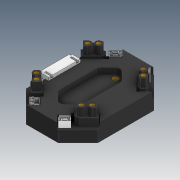
# Autodesk Inventor part: terminal_board
Saved by Autodesk Inventor 2020 (Build 240168000, 168)
## iProperties
Created: 2020-09-28
Part Number: terminal_board
Material: Generic
Document SubType Name: Modeling
Designer: DELL
Density: 1 g/cm^3
Appearance: White
Author: DELL
Autodesk Inventor part; units mm, degrees
ref_plane "YZ Plane" through (0, 0, 0) normal (1, 0, 0) x (0, 1, 0)
ref_plane "XZ Plane" through (0, 0, 0) normal (0, 1, 0) x (-1, 0, 0)
ref_plane "XY Plane" through (0, 0, 0) normal (0, 0, 1) x (1, 0, 0)
sketch "Sketch1" plane through (0, 0, 0) normal (0, 1, 0) x (-1, 0, 0)
  line L0 (22.5, 17.5) -> (22.5, -17.5)
  line L1 (22.5, -17.5) -> (10, -30)
  line L2 (10, -30) -> (-10, -30)
  line L3 (-10, -30) -> (-22.5, -17.5)
  line L4 (-22.5, -17.5) -> (-22.5, 17.5)
  line L5 (-22.5, 17.5) -> (-10, 30)
  line L6 (-10, 30) -> (10, 30)
  line L7 (10, 30) -> (22.5, 17.5)
  line L8 (30.1038, 0) -> (-31.33, 0) construction
  line L9 (0, 32.2243) -> (0, -47.739) construction
  point P0 (0, 0)
  dimension "d0" = 45
  dimension "d1" = 60
  dimension "d2" = 20
  dimension "d3" = 35
  constraints: 20 end point, 2 horizontal, 2 point on line, 2 vertical, 1 parallel, 1 perpendicular, 5 other
  measures "d0" distance between parallel lines of L4 L0
  measures "d1" distance between parallel lines of L2 L6
  measures "d2" distance of L1.end L2.end
  measures "d3" distance of L0.start L0.end
extrude "Extrusion1" add sketch "Sketch1" along normal blind 6.8
sketch "Sketch2" plane through (0, 6.8, 0) normal (0, 1, 0) x (1, 0, 0)
  line L0 (-21.4393, 15.7322) -> (-15.4289, 21.7426)
  line L1 (-15.4289, 21.7426) -> (-11.6813, 17.995)
  line L2 (-11.6813, 17.995) -> (-17.6917, 11.9846)
  line L3 (-17.6917, 11.9846) -> (-21.4393, 15.7322)
  line L4 (-10, 30) -> (-22.5, 17.5) projected
  line L5 (-15.4289, 21.7426) -> (-12.6712, 22.5205)
  line L6 (-12.6712, 22.5205) -> (-10.9034, 20.7527)
  line L7 (-10.9034, 20.7527) -> (-11.6813, 17.995)
  line L8 (-19.5655, 13.8584) -> (-13.5551, 19.8688) construction
  point P0 (0, 0)
  dimension "d6" = 5.3
  dimension "d7" = 11
  dimension "d8" = 8.5
  dimension "d9" = 2.5
  dimension "d10" = 2
  dimension "d11" = 0.5
  constraints: 17 end point, 3 perpendicular, 2 midpoint, 1 parallel, 1 other
  measures "d6" distance between parallel lines of L2 L0
  measures "d7" distance between parallel lines of L3 L6
  measures "d8" distance between parallel lines of L3 L1
  measures "d9" distance of L5.end L6.end
  measures "d10" distance between parallel lines of L4 L0
  measures "d11" distance from line of L4.end L3
extrude "Extrusion2" add sketch "Sketch2" along normal blind 5.2
sketch "Sketch3" plane through (0, 12, 0) normal (0, 1, 0) x (1, 0, 0)
  line L0 (-10.9034, 20.7527) -> (-12.6712, 22.5205) projected
  line L1 (-12.6712, 22.5205) -> (-15.4289, 21.7426) projected
  line L2 (-15.4289, 21.7426) -> (-21.4393, 15.7322) projected
  line L3 (-21.4393, 15.7322) -> (-17.6917, 11.9846) projected
  line L4 (-17.6917, 11.9846) -> (-11.6813, 17.995) projected
  line L5 (-11.6813, 17.995) -> (-10.9034, 20.7527) projected
  line L6 (-14.5509, 21.4708) -> (-13.3632, 21.8058)
  circle A0 centre (-17.3735, 16.0504) radius 1.25
  circle A1 centre (-13.9794, 19.4445) radius 1.25
  line L7 (-19.212, 14.212) -> (-12.1409, 21.283) construction
  line L8 (-17.1967, 19.2678) -> (-14.1561, 16.2272) construction
  line L9 (-17.3735, 13.0731) -> (-15.8848, 14.5618)
  line L10 (-17.3735, 13.0731) -> (-20.3508, 16.0504)
  line L11 (-13.3632, 21.8058) -> (-11.6181, 20.0607)
  line L12 (-10.9034, 20.7527) -> (-12.6712, 22.5205) projected
  line L13 (-15.7186, 17.3518) -> (-15.2807, 17.7896)
  line L14 (-16.0721, 17.7053) -> (-15.6343, 18.1432)
  line L15 (-11.6181, 20.0607) -> (-11.9531, 18.873)
  line L16 (-20.3508, 16.0504) -> (-18.8621, 17.5391)
  arc A2 (-15.8848, 14.5618) -> (-15.7186, 17.3518) centre (-17.3735, 16.0504) ccw
  arc A3 (-16.0721, 17.7053) -> (-18.8621, 17.5391) centre (-17.3735, 16.0504) ccw
  arc A4 (-14.5509, 21.4708) -> (-15.6343, 18.1432) centre (-13.9794, 19.4445) ccw
  arc A5 (-15.2807, 17.7896) -> (-11.9531, 18.873) centre (-13.9794, 19.4445) ccw
  point P0 (0, 0)
  dimension "d15" = 4.8
  dimension "d16" = 2.5
  dimension "d17" = 0.5
  constraints: 20 end point, 8 point on circle, 6 centre point, 5 tangent, 2 coincident, 2 parallel, 2 point on line, 1 equal radius, 1 symmetric about line, 1 other
  measures "d15" distance of A1.centre A0.centre
  measures "d16" diameter of A0
  measures "d17" distance between parallel lines of L13 L14
extrude "Extrusion3" add sketch "Sketch3" along normal blind 5.2 contours L6 L11 L15 A5 L13 A2 L9 L10 L16 A3 L14 A4
sketch "Sketch4" plane through (0, 6.8, 0) normal (0, 1, 0) x (1, 0, 0)
  line L0 (-15.7186, 17.3518) -> (-15.2807, 17.7896) projected
  line L1 (-15.4996, 17.5707) -> (0, 2.0711)
  line L2 (0, 0) -> (0, 30.0261)
  constraints: 4 end point, 1 coincident, 1 midpoint, 1 perpendicular, 1 point on line, 1 vertical
fillet "Fillet1" radius 0.2 4 edges at (-15.7186, 14.6, -17.3518) (-15.2807, 14.6, -17.7896) (-16.0721, 14.6, -17.7053) (-15.6343, 14.6, -18.1432)
fillet "Fillet2" radius 0.2 2 edges at (-11.6181, 14.6, -20.0607) (-13.3632, 14.6, -21.8058)
pattern_circular "Circular Pattern1" count 2 over 270 about axis through (0, 6.8, -2.0711) along (0, 1, 0) of "Extrusion2", "Extrusion3", "Fillet1", "Fillet2"
pattern_circular "Circular Pattern2" count 2 over 360 about axis through (0, -10, 0) along (0, 1, 0) of "Extrusion2", "Extrusion3", "Fillet1", "Fillet2", "Circular Pattern1"
sketch "Sketch5" plane through (0, 6.8, 0) normal (0, 1, 0) x (1, 0, 0)
  line L0 (-13.0406, 24.8381) -> (-9.8586, 21.6561)
  line L1 (-9.8586, 21.6561) -> (-5.7574, 25.7574)
  line L2 (-5.7574, 25.7574) -> (-8.9393, 28.9393)
  line L3 (-8.9393, 28.9393) -> (-13.0406, 24.8381)
  line L4 (-10, 30) -> (-22.5, 17.5) projected
  line L5 (10, 30) -> (-10, 30) projected
  point P0 (0, 0)
  point P1 (-10, 30)
  dimension "d28" = 1.5
  dimension "d29" = 5.8
  dimension "d30" = 4.5
  constraints: 8 end point, 2 parallel, 2 perpendicular, 1 coincident, 1 point on line
  measures "d28" distance between parallel lines of L4 L3
  measures "d29" distance of L2.end L0.start
  measures "d30" distance of L1.end L2.end
extrude "Extrusion4" add sketch "Sketch5" along normal blind 4.15
sketch "Sketch6" plane through (0, 10.95, 0) normal (0, 1, 0) x (1, 0, 0)
  line L0 (-12.6163, 24.8381) -> (-12.192, 24.4139)
  line L1 (-12.192, 24.4139) -> (-11.4849, 25.121)
  line L2 (-11.4849, 25.121) -> (-11.9092, 25.5452)
  line L3 (-11.9092, 25.5452) -> (-12.6163, 24.8381)
  line L4 (-8.9393, 28.9393) -> (-13.0406, 24.8381) projected
  line L5 (-13.0406, 24.8381) -> (-9.8586, 21.6561) projected
  line L6 (-13.0406, 24.8381) -> (-8.9393, 28.9393) construction
  line L7 (-10.9899, 26.8887) -> (-7.808, 23.7067) construction
  line L8 (-8.9393, 28.5151) -> (-8.5151, 28.0908)
  line L9 (-8.5151, 28.0908) -> (-9.2222, 27.3837)
  line L10 (-9.2222, 27.3837) -> (-9.6464, 27.808)
  line L11 (-9.6464, 27.808) -> (-8.9393, 28.5151)
  line L12 (-11.5556, 25.8988) -> (-10.4243, 24.7674)
  line L13 (-10.4243, 24.7674) -> (-8.8686, 26.323)
  line L14 (-8.8686, 26.323) -> (-10, 27.4544)
  line L15 (-10, 27.4544) -> (-11.5556, 25.8988)
  line L16 (-5.7574, 25.7574) -> (-8.9393, 28.9393) construction
  line L17 (-8.9393, 28.9393) -> (-13.0406, 24.8381) construction
  line L18 (-13.0406, 24.8381) -> (-9.8586, 21.6561) construction
  line L19 (-9.8586, 21.6561) -> (-5.7574, 25.7574) construction
  line L20 (-8.9393, 28.5151) -> (-12.6163, 24.8381) construction
  line L21 (-9.6464, 22.2925) -> (-6.3938, 25.5452)
  line L22 (-11.7678, 24.4139) -> (-11.1314, 25.0503)
  line L23 (-11.1314, 25.0503) -> (-10.4243, 24.3431)
  line L24 (-10.4243, 24.3431) -> (-8.4444, 26.323)
  line L25 (-8.4444, 26.323) -> (-9.1515, 27.0302)
  line L26 (-9.1515, 27.0302) -> (-8.5151, 27.6665)
  line L27 (-12.6163, 24.8381) -> (-12.192, 24.4139)
  line L28 (-11.7678, 24.4139) -> (-9.6464, 22.2925)
  line L29 (-6.3938, 25.5452) -> (-8.5151, 27.6665)
  line L30 (-8.5151, 28.0908) -> (-8.9393, 28.5151)
  point P0 (0, 0)
  dimension "d34" = 0.3
  dimension "d35" = 0.3
  dimension "d36" = 1
  dimension "d37" = 0.6
  dimension "d40" = 2.2
  dimension "d41" = 1.6
  dimension "d42" = 0.3
  dimension "d43" = 0.3
  dimension "d45" = 0.3
  dimension "d46" = 0.3
  dimension "d47" = 0.3
  dimension "d48" = 0.6
  dimension "d49" = 0.6
  dimension "d50" = 0.3
  constraints: 48 end point, 10 perpendicular, 4 symmetric about line, 2 point on line, 1 midpoint, 1 parallel, 1 other
  measures "d34" distance between parallel lines of L4 L3
  measures "d35" distance between parallel lines of L5 L0
  measures "d36" distance of L0.end L1.end
  measures "d37" distance of L0.start L0.end
  measures "d40" distance of L14.end L12.start
  measures "d41" distance of L12.start L12.end
  measures "d42" distance between parallel lines of L4 L15
  measures "d43" distance between parallel lines of L12 L23
  measures "d45" distance between parallel lines of L13 L24
  measures "d46" distance between parallel lines of L14 L25
  measures "d47" distance between parallel lines of L9 L26
  measures "d48" distance between parallel lines of L5 L28
  measures "d49" distance between parallel lines of L16 L29
  measures "d50" distance between parallel lines of L19 L21
extrude "Extrusion5" cut sketch "Sketch6" against normal up to surface (4.15 mm away) contours L3 L2 L1 L0 | L8 L9 L10 L11 | L15 L14 L13 L12
extrude "Extrusion6" cut sketch "Sketch6" against normal blind 3 contours L28 L22 L23 L24 L25 L26 L29 L21
sketch "Sketch7" plane through (-8.9393, 6.8, -28.9393) normal (0.7071068, 0, -0.7071068) x (-0.7071068, 0, -0.7071068)
  line L0 (-4.5, 4.15) -> (0, 4.15) projected
  line L1 (-1.9, 4.15) -> (-4.5, 4.15)
  line L2 (-4.5, 4.15) -> (-4.5, 1.8317)
  line L3 (-4.5, 0) -> (-4.5, 4.15) projected
  line L4 (-4.5, 1.8317) -> (-3.7, 1.8317)
  line L5 (-3.7, 1.8317) -> (-3.7, 3.55)
  line L6 (-3.7, 3.55) -> (-1.9, 3.55)
  line L7 (-1.9, 4.15) -> (-1.9, 0) projected
  line L8 (-1.9, 3.55) -> (-1.9, 4.15)
  point P0 (-26.7843, -6.8)
  dimension "d55" = 0.6
  dimension "d56" = 0.8
  constraints: 12 end point, 3 perpendicular, 3 point on line, 1 collinear, 1 horizontal
  measures "d55" distance between parallel lines of L0 L6
  measures "d56" distance between parallel lines of L5 L2
extrude "Extrusion7" cut sketch "Sketch7" against normal blind 0.3
ref_plane "Work Plane1" through (-10.9899, 6.8, -26.8887) normal (0.7071068, 0, -0.7071068) x (-0.7071068, 0, -0.7071068)
mirror "Mirror1" about plane through (-10.9899, 6.8, -26.8887) normal (0.7071068, 0, -0.7071068) of "Extrusion7"
sketch "Sketch8" plane through (0, 6.8, 0) normal (0, 1, 0) x (1, 0, 0)
  line L0 (0, 0) -> (0, 30)
  line L1 (10, 30) -> (-10, 30) projected
  line L2 (-8.9393, 28.9393) -> (-13.0406, 24.8381) projected
  line L3 (-10.9899, 26.8887) -> (0, 15.8988)
  constraints: 4 end point, 2 midpoint, 1 coincident, 1 perpendicular, 1 point on line
pattern_circular "Circular Pattern3" count 2 over 270 about axis through (0, 6.8, -15.8988) along (0, 1, 0) of "Extrusion6", "Extrusion4", "Extrusion5", "Extrusion7", "Mirror1"
pattern_circular "Circular Pattern4" count 2 over 360 about axis through (0, -10, 0) along (0, 1, 0) of "Extrusion4", "Extrusion5", "Extrusion6", "Extrusion7", "Mirror1", "Circular Pattern3"
sketch "Sketch9" plane through (0, 6.8, 0) normal (0, 1, 0) x (1, 0, 0)
  line L0 (-16, -10) -> (-22, -10)
  line L1 (-22, -10) -> (-22, 10)
  line L2 (-22, 10) -> (-16, 10)
  line L3 (-16, 10) -> (-16, -10)
  line L4 (-16, -10) -> (-22, 10) construction
  line L5 (-22, -10) -> (-16, 10) construction
  line L6 (-22.5, 17.5) -> (-22.5, -17.5) projected
  line L7 (-22.5, 0) -> (22.5, 0) construction
  line L8 (22.5, -17.5) -> (22.5, 17.5) construction
  point P0 (0, 0)
  point P1 (-19, 0)
  point P2 (-19, 0)
  dimension "d65" = 20
  dimension "d66" = 6
  dimension "d67" = 0.5
  constraints: 14 end point, 5 midpoint, 2 parallel, 1 horizontal, 1 perpendicular, 1 point on line
  measures "d65" distance of L0.end L1.end
  measures "d66" distance of L1.end L2.end
  measures "d67" distance between parallel lines of L6 L1
extrude "Extrusion8" add sketch "Sketch9" along normal blind 5.6
sketch "Sketch10" plane through (-22, 6.8, -10) normal (-1, 0, 0) x (0, 0, 1)
  line L0 (20, 0) -> (0, 0) projected
  line L1 (20, 0) -> (20, 5.6) projected
  line L2 (0, 5.6) -> (20, 5.6) projected
  line L3 (0, 0) -> (0, 5.6) projected
  line L4 (19.5, 4.36) -> (19.5, 0.5)
  line L5 (19.5, 0.5) -> (0.5, 0.5)
  line L6 (0.5, 0.5) -> (0.5, 4.36)
  line L7 (4, 5.1) -> (16, 5.1)
  line L8 (0.5, 4.36) -> (0.5, 0.5)
  line L9 (0.5, 0.5) -> (19.5, 0.5)
  line L10 (19.5, 0.5) -> (19.5, 4.36)
  line L11 (19.5, 4.36) -> (0.5, 0.5) construction
  line L12 (0.5, 4.36) -> (19.5, 0.5) construction
  line L13 (4, 4.36) -> (4, 5.1)
  line L14 (4, 5.1) -> (16, 5.1)
  line L15 (16, 5.1) -> (16, 4.36)
  line L16 (16, 4.36) -> (4, 5.1) construction
  line L17 (4, 4.36) -> (16, 5.1) construction
  line L18 (19.5, 4.36) -> (16, 4.36)
  line L19 (4, 4.36) -> (0.5, 4.36)
  point P0 (10, -6.8)
  point P1 (10, 2.43)
  point P2 (10, 4.73)
  point P3 (10, 4.73)
  point P4 (10, 2.43)
  dimension "d70" = 0.5
  dimension "d72" = 12
  dimension "d73" = 3.86
  dimension "d74" = 19
  dimension "d75" = 0.5
  dimension "d76" = 4.36
  constraints: 32 end point, 6 midpoint, 4 parallel, 3 collinear, 2 horizontal, 2 perpendicular, 1 vertical alignment
  measures "d70" distance between parallel lines of L2 L7
  measures "d72" distance of L7.start L7.end
  measures "d73" distance between parallel lines of L5 L19
  measures "d74" distance between parallel lines of L4 L6
  measures "d75" distance between parallel lines of L3 L6
  measures "d76" distance between parallel lines of L0 L19
extrude "Extrusion9" cut sketch "Sketch10" against normal blind 5.6 contours L4 L5 L6 L19 L13 L7 L15 L18
sketch "Sketch11" plane through (0, 12.4, 0) normal (0, 1, 0) x (1, 0, 0)
  line L0 (-16, 8.5) -> (-20, 8.5)
  line L1 (-20, 8.5) -> (-20, 7.5)
  line L2 (-20, 7.5) -> (-16, 7.5)
  line L3 (-16, 7.5) -> (-16, 8.5)
  line L4 (-16, 10) -> (-16, -10) projected
  line L5 (-16, -7.5) -> (-20, -7.5)
  line L6 (-20, -7.5) -> (-20, -8.5)
  line L7 (-20, -8.5) -> (-16, -8.5)
  line L8 (-16, -8.5) -> (-16, -7.5)
  line L9 (-16, 10) -> (-22, 10) projected
  line L10 (-22, 10) -> (-22, -10) projected
  line L11 (-16, 0) -> (-22, 0) construction
  line L12 (-22, 6) -> (-22, -6) construction
  point P0 (0, 0)
  dimension "d79" = 1
  dimension "d80" = 1.5
  dimension "d81" = 2
  constraints: 18 end point, 4 parallel, 2 horizontal, 2 midpoint, 2 perpendicular, 2 point on line, 2 other
  measures "d79" distance of L0.end L1.end
  measures "d80" distance between parallel lines of L9 L0
  measures "d81" distance between parallel lines of L10 L1
extrude "Extrusion10" cut sketch "Sketch11" against normal up to surface (1.24 mm away)
sketch "Sketch12" plane through (0, 12.4, 0) normal (0, 1, 0) x (1, 0, 0)
  line L0 (-16, 10) -> (-22, 10) projected
  line L1 (-22, 10) -> (-21, 10)
  line L2 (-21, 10) -> (-21, 9)
  line L3 (-21, 9) -> (-22, 9)
  line L4 (-22, 9) -> (-22, 10)
  line L5 (-22, -10) -> (-16, -10) projected
  line L6 (-22, -10) -> (-21, -10)
  line L7 (-21, -10) -> (-21, -9)
  line L8 (-21, -9) -> (-22, -9)
  line L9 (-22, -9) -> (-22, -10)
  point P0 (0, 0)
  dimension "d84" = 1
  dimension "d85" = 1
  dimension "d86" = 1
  dimension "d87" = 1
  constraints: 16 end point, 4 parallel, 2 horizontal, 2 perpendicular
  measures "d84" distance of L2.end L3.end
  measures "d85" distance of L1.end L2.end
  measures "d86" distance of L7.end L8.end
  measures "d87" distance of L6.end L7.end
extrude "Extrusion11" cut sketch "Sketch12" against normal up to surface (5.6 mm away)
sketch "Sketch13" plane through (-21, 12.4, 9) normal (-1, 0, 0) x (0, 0, 1)
  line L0 (-19, -5.6) -> (-19, 0) projected
  line L1 (1, -2.5) -> (-19, -2.5)
  line L2 (-19, -2.5) -> (-19, -2)
  line L3 (-19, -2) -> (1, -2)
  line L4 (1, -2) -> (1, -2.5)
  line L5 (1, -2.5) -> (-19, -2) construction
  line L6 (-19, -2.5) -> (1, -2) construction
  line L7 (-18, 0) -> (0, 0) projected
  line L8 (1, 0) -> (1, -5.6) projected
  point P0 (-9, -12.4)
  point P1 (-9, -2.25)
  dimension "d90" = 2
  dimension "d91" = 0.5
  constraints: 12 end point, 2 midpoint, 2 parallel, 1 collinear, 1 horizontal, 1 perpendicular, 1 point on line
  measures "d90" distance between parallel lines of L7 L3
  measures "d91" distance between parallel lines of L1 L3
extrude "Extrusion12" cut sketch "Sketch13" against normal blind 1.5
sketch "Sketch14" plane through (0, 6.8, 0) normal (0, 1, 0) x (1, 0, 0)
  line L0 (-16, -10) -> (-21, -10) projected
  line L1 (-21, -9) -> (-21, -10) projected
  line L2 (-22, -9) -> (-21, -9) projected
  line L3 (-22, -9) -> (-22, 9) projected
  line L4 (-21, 9) -> (-22, 9) projected
  line L5 (-21, 10) -> (-21, 9) projected
  line L6 (-21, 10) -> (-16, 10) projected
  line L7 (-16, 10) -> (-16, -10) projected
  line L8 (-5.7574, -25.7574) -> (-8.9393, -28.9393) projected
  line L9 (-8.9393, -28.9393) -> (-13.0406, -24.8381) projected
  line L10 (-13.0406, -24.8381) -> (-9.8586, -21.6561) projected
  line L11 (-9.8586, -21.6561) -> (-5.7574, -25.7574) projected
  line L12 (9.8586, -21.6561) -> (13.0406, -24.8381) projected
  line L13 (13.0406, -24.8381) -> (8.9393, -28.9393) projected
  line L14 (8.9393, -28.9393) -> (5.7574, -25.7574) projected
  line L15 (5.7574, -25.7574) -> (9.8586, -21.6561) projected
  line L16 (5.7574, 25.7574) -> (8.9393, 28.9393) projected
  line L17 (8.9393, 28.9393) -> (13.0406, 24.8381) projected
  line L18 (13.0406, 24.8381) -> (9.8586, 21.6561) projected
  line L19 (9.8586, 21.6561) -> (5.7574, 25.7574) projected
  line L20 (-9.8586, 21.6561) -> (-13.0406, 24.8381) projected
  line L21 (-13.0406, 24.8381) -> (-8.9393, 28.9393) projected
  line L22 (-8.9393, 28.9393) -> (-5.7574, 25.7574) projected
  line L23 (-5.7574, 25.7574) -> (-9.8586, 21.6561) projected
  line L24 (-9.9135, -19.7627) -> (-13.6612, -23.5104) projected
  line L25 (-13.6612, -23.5104) -> (-19.6716, -17.5) projected
  line L26 (-19.6716, -17.5) -> (-20.4494, -14.7423) projected
  line L27 (-20.4494, -14.7423) -> (-18.6816, -12.9745) projected
  line L28 (-18.6816, -12.9745) -> (-15.9239, -13.7523) projected
  line L29 (-15.9239, -13.7523) -> (-9.9135, -19.7627) projected
  line L30 (17.6917, -11.9846) -> (21.4393, -15.7322) projected
  line L31 (21.4393, -15.7322) -> (15.4289, -21.7426) projected
  line L32 (15.4289, -21.7426) -> (12.6712, -22.5205) projected
  line L33 (12.6712, -22.5205) -> (10.9034, -20.7527) projected
  line L34 (10.9034, -20.7527) -> (11.6813, -17.995) projected
  line L35 (11.6813, -17.995) -> (17.6917, -11.9846) projected
  line L36 (9.9135, 19.7627) -> (13.6612, 23.5104) projected
  line L37 (13.6612, 23.5104) -> (19.6716, 17.5) projected
  line L38 (19.6716, 17.5) -> (20.4494, 14.7423) projected
  line L39 (20.4494, 14.7423) -> (18.6816, 12.9745) projected
  line L40 (18.6816, 12.9745) -> (15.9239, 13.7523) projected
  line L41 (15.9239, 13.7523) -> (9.9135, 19.7627) projected
  line L42 (-17.6917, 11.9846) -> (-21.4393, 15.7322) projected
  line L43 (-21.4393, 15.7322) -> (-15.4289, 21.7426) projected
  line L44 (-15.4289, 21.7426) -> (-12.6712, 22.5205) projected
  line L45 (-12.6712, 22.5205) -> (-10.9034, 20.7527) projected
  line L46 (-10.9034, 20.7527) -> (-11.6813, 17.995) projected
  line L47 (-11.6813, 17.995) -> (-17.6917, 11.9846) projected
  line L48 (-10, -30) -> (10, -30) projected
  line L49 (10, -30) -> (22.5, -17.5) projected
  line L50 (22.5, -17.5) -> (22.5, 17.5) projected
  line L51 (22.5, 17.5) -> (10, 30) projected
  line L52 (10, 30) -> (-10, 30) projected
  line L53 (-10, 30) -> (-22.5, 17.5) projected
  line L54 (-22.5, 17.5) -> (-22.5, -17.5) projected
  line L55 (-22.5, -17.5) -> (-10, -30) projected
  line L56 (14.9, -14.352) -> (8.7272, -20.5248)
  line L57 (-8.7272, -20.5248) -> (-14.9, -14.352)
  line L58 (-14.9, 14.352) -> (-8.7272, 20.5248)
  line L59 (8.7272, 20.5248) -> (14.9, 14.352)
  line L60 (-14.9, 14.352) -> (-17.9, 11.352)
  line L61 (-11.6813, 17.995) -> (-17.6917, 11.9846) projected
  line L62 (-17.9, 11.352) -> (-17.9, 10.3)
  line L63 (-17.9, 10.3) -> (-15.7, 10.3)
  line L64 (-15.7, 10.3) -> (-15.7, 0)
  line L65 (22.5, 0) -> (-22.5, 0) construction
  line L66 (10, 30) -> (-10, 30) construction
  line L67 (0, 30) -> (0, -30) construction
  line L68 (-14.9, -14.352) -> (-17.9, -11.352)
  line L69 (-17.9, -11.352) -> (-17.9, -10.3)
  line L70 (-17.9, -10.3) -> (-15.7, -10.3)
  line L71 (-15.7, -10.3) -> (-15.7, 0)
  line L72 (-8.7272, -20.5248) -> (-9.6464, -21.444)
  line L73 (-9.8586, -21.6561) -> (-5.7574, -25.7574) projected
  line L74 (-9.6464, -21.444) -> (-5.3331, -25.7574)
  line L75 (-5.3331, -25.7574) -> (-9.5757, -30)
  line L76 (-10, -30) -> (10, -30) projected
  line L77 (-9.5757, -30) -> (0, -30)
  line L78 (9.5757, -30) -> (-9.5757, -30)
  line L79 (8.7272, -20.5248) -> (9.6464, -21.444)
  line L80 (9.6464, -21.444) -> (5.3331, -25.7574)
  line L81 (5.3331, -25.7574) -> (9.5757, -30)
  line L82 (14.9, -14.352) -> (17.6917, -11.5603)
  line L83 (17.6917, -11.5603) -> (22.5, -16.3686)
  line L84 (22.5, -16.3686) -> (22.5, 16.3686)
  line L85 (22.5, -17.5) -> (22.5, 17.5) projected
  line L86 (22.5, 16.3686) -> (17.6917, 11.5603)
  line L87 (17.6917, 11.5603) -> (14.9, 14.352)
  line L88 (-10, 30) -> (10, 30)
  line L89 (-8.7272, 20.5248) -> (-9.6464, 21.444)
  line L90 (-9.6464, 21.444) -> (-5.3331, 25.7574)
  line L91 (-5.3331, 25.7574) -> (-9.5757, 30)
  line L92 (8.7272, 20.5248) -> (9.6464, 21.444)
  line L93 (9.6464, 21.444) -> (5.3331, 25.7574)
  line L94 (5.3331, 25.7574) -> (9.5757, 30)
  point P0 (0, 0)
  point P1 (10, -30)
  point P2 (-10, -30)
  point P3 (-14.9, 10.3)
  point P4 (22.5, 16.3686)
  dimension "d95" = 0.3
  dimension "d97" = 0.3
  dimension "d98" = 0.3
  dimension "d99" = 0.3
  dimension "d100" = 0.3
  dimension "d101" = 0.3
  constraints: 68 end point, 19 symmetric about line, 5 perpendicular, 4 midpoint, 3 point on line, 2 collinear, 2 parallel, 1 vertical
  measures "d95" distance between parallel lines of L6 L63
  measures "d97" distance between parallel lines of L7 L64
  measures "d98" distance between parallel lines of L11 L74
  measures "d99" distance between parallel lines of L8 L75
  measures "d100" distance between parallel lines of L30 L83
  measures "d101" distance between parallel lines of L39 L86
extrude "Extrusion13" add sketch "Sketch14" along normal blind 4 contours L75 L74 L72 L57 L68 L69 L70 L71 L64 L63 L62 L60 L58 L89 L90 L91 L52 L94 L93 L92 L59 L87 L86 L50 L83 L82 L56 L79 L80 L81 L48
sketch "Sketch15" plane through (0, 10.8, 0) normal (0, 1, 0) x (1, 0, 0)
  line L0 (-7.5, -12.5) -> (7.5, -12.5)
  line L1 (7.5, -12.5) -> (7.5, 12.5)
  line L2 (7.5, 12.5) -> (-7.5, 12.5)
  line L3 (-7.5, 12.5) -> (-7.5, -12.5)
  line L4 (-7.5, -12.5) -> (7.5, 12.5) construction
  line L5 (7.5, -12.5) -> (-7.5, 12.5) construction
  line L6 (7.5, 12.5) -> (0, 20)
  line L7 (0, 20) -> (-7.5, 12.5)
  line L8 (7.5, -12.5) -> (0, -20)
  line L9 (0, -20) -> (-7.5, -12.5)
  line L10 (9.5757, 30) -> (-9.5757, 30) construction
  line L11 (0, 30) -> (0, -30) construction
  line L12 (-10, -30) -> (10, -30) construction
  point P0 (0, 0)
  dimension "d104" = 15
  dimension "d105" = 25
  constraints: 22 end point, 4 midpoint, 4 parallel, 2 perpendicular, 1 horizontal, 1 point on line
  measures "d104" distance between parallel lines of L3 L1
  measures "d105" distance of L2.end L0.start
extrude "Extrusion14" cut sketch "Sketch15" against normal blind 4
fillet "Fillet3" radius 3 6 edges at (7.5, 8.8, -12.5) (7.5, 8.8, 12.5) (-7.5, 8.8, 12.5) (-7.5, 8.8, -12.5) (0, 8.8, -20) (0, 8.8, 20)
sketch "Sketch16" plane through (0, 6.8, 0) normal (0, 1, 0) x (1, 0, 0)
  circle A0 centre (0, -16) radius 1.75
  circle A1 centre (0, 16) radius 1.75
  line L0 (7.5, 11.2574) -> (7.5, -11.2574) construction
  line L1 (7.5, 0) -> (-7.5, 0) construction
  line L2 (-7.5, -11.2574) -> (-7.5, 11.2574) construction
  point P0 (0, 0)
  dimension "d109" = 32
  dimension "d110" = 3.5
  constraints: 2 centre point, 2 end point, 2 midpoint, 1 equal radius, 1 symmetric about line
  measures "d109" distance of A1.centre A0.centre
  measures "d110" diameter of A1
extrude "Extrusion15" cut sketch "Sketch16" against normal through all
body "Solid1"
